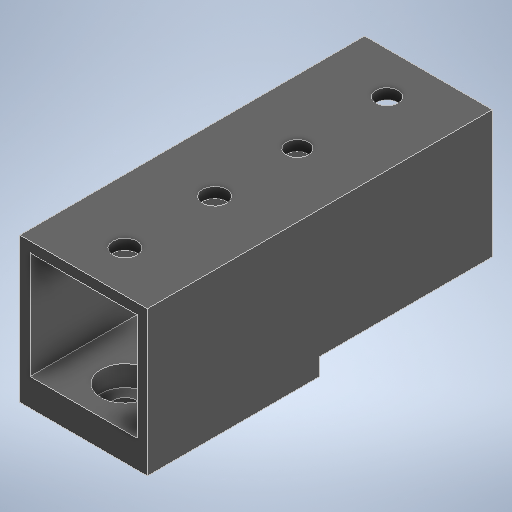
# Autodesk Inventor part: pole_setter_arm
Saved by Autodesk Inventor 2026.1 (Build 301233020, 233B)
## iProperties
Created: 2026-02-01
Part Number: pole_setter_arm
Material: 一般
Document SubType Name: Modeling
Designer: hibik
Density: 1 g/cm^3
Appearance: 既定
Author: hibik
Autodesk Inventor part; units mm, degrees
ref_plane "YZ Plane" through (0, 0, 0) normal (1, 0, 0) x (0, 1, 0)
ref_plane "XZ Plane" through (0, 0, 0) normal (0, 1, 0) x (-1, 0, 0)
ref_plane "XY Plane" through (0, 0, 0) normal (0, 0, 1) x (1, 0, 0)
sketch "スケッチ1" plane through (0, 0, 0) normal (0, 1, 0) x (-1, 0, 0)
  line L0 (0, 12.5) -> (18.5, 12.5)
  line L1 (18.5, 12.5) -> (18.5, -12.5)
  line L2 (18.5, -12.5) -> (0, -12.5)
  line L3 (0, -12.5) -> (0, 12.5)
  point P0 (0, 0)
  point P1 (0, 0)
  dimension "d0" = 18.5
  dimension "d1" = 25
  constraints: 8 end point, 2 parallel, 1 coincident, 1 horizontal, 1 midpoint, 1 perpendicular
  measures "d0" distance of L1.end L2.end
  measures "d1" distance of L0.end L1.end
extrude "押し出し1" add sketch "スケッチ1" along normal blind 1
sketch "スケッチ3" plane through (0, 1, 0) normal (0, 1, 0) x (1, 0, 0)
  circle A0 centre (-9.25, -6.5) radius 1.75
  circle A1 centre (-9.25, 6.5) radius 1.75
  line L0 (-22.2, 0) -> (3.7, 0) projected
  line L1 (-18.5, -12.5) -> (0, -12.5) projected
  point P0 (0, 0)
  point P1 (-9.25, -12.5)
  dimension "d9" = 6
  dimension "d10" = 3.5
  constraints: 2 centre point, 1 midpoint, 1 vertical alignment, 1 other
  measures "d9" distance from line of L1 A0.centre
  measures "d10" diameter of A0
extrude "押し出し3" cut sketch "スケッチ3" against normal through all
sketch "スケッチ4" plane through (0, 1, 0) normal (0, 1, 0) x (1, 0, 0)
  circle A0 centre (-9.25, -6.5) radius 1.75 projected
  circle A1 centre (-9.25, 6.5) radius 1.75 projected
  line L0 (0, 12.5) -> (-18.5, 12.5) projected
  line L1 (-18.5, 12.5) -> (-18.5, -12.5) projected
  line L2 (-18.5, -12.5) -> (0, -12.5) projected
  line L3 (0, -12.5) -> (0, 12.5) projected
  circle A2 centre (-9.25, 6.5) radius 3.5
  circle A3 centre (-9.25, -6.5) radius 3.5
  point P0 (0, 0)
  dimension "d13" = 7
  dimension "d14" = 7
  constraints: 2 centre point, 2 coincident
  measures "d13" diameter of A2
  measures "d14" diameter of A3
extrude "押し出し4" add sketch "スケッチ4" along normal blind 1.5 contours L3 L2 L1 L0
sketch "スケッチ5" plane through (-18.5, 0, 12.5) normal (0, 0, 1) x (1, 0, 0)
  line L0 (0, 2.5) -> (18.5, 2.5)
  line L1 (18.5, 2.5) -> (18.5, 21)
  line L2 (18.5, 21) -> (0, 21)
  line L3 (0, 21) -> (0, 2.5)
  line L4 (1.5, 4) -> (17, 4)
  line L5 (17, 4) -> (17, 19.5)
  line L6 (17, 19.5) -> (1.5, 19.5)
  line L7 (1.5, 19.5) -> (1.5, 4)
  point P0 (18.5, 0)
  point P1 (9.25, 19.5)
  point P2 (9.25, 21)
  dimension "d17" = 1.5
  dimension "d18" = 1.5
  dimension "d19" = 15.5
  constraints: 16 end point, 4 parallel, 4 perpendicular, 2 horizontal, 2 midpoint, 1 coincident, 1 vertical alignment
  measures "d17" distance between parallel lines of L2 L6
  measures "d18" distance between parallel lines of L7 L3
  measures "d19" distance of L4.end L5.end
extrude "押し出し5" add sketch "スケッチ5" against normal up to surface (25 mm away)
sketch "スケッチ6" plane through (-17, 4, 12.5) normal (0, 1, 0) x (1, 0, 0)
  circle A0 centre (7.75, 6) radius 3.5 projected
  circle A1 centre (7.75, 19) radius 3.5 projected
  point P0 (17, 12.5)
extrude "押し出し6" cut sketch "スケッチ6" against normal up to surface (1.5 mm away)
sketch "スケッチ7" plane through (-18.5, 21, 12.5) normal (0, 1, 0) x (1, 0, 0)
  circle A0 centre (9.25, 19) radius 1.75 projected
  circle A1 centre (9.25, 6) radius 1.75 projected
  point P0 (18.5, 12.5)
extrude "押し出し7" cut sketch "スケッチ7" against normal through all
sketch "スケッチ9" plane through (0, 0, -12.5) normal (0, 0, -1) x (-1, 0, 0)
  line L0 (0, 0) -> (0, 21) projected
  line L1 (18.5, 0) -> (18.5, 21) projected
  line L2 (0, 2.5) -> (18.5, 2.5)
  line L3 (18.5, 2.5) -> (18.5, 21)
  line L4 (18.5, 21) -> (0, 21)
  line L5 (0, 21) -> (0, 2.5)
  line L6 (1.5, 4) -> (17, 4) projected
  line L7 (1.5, 19.5) -> (1.5, 4) projected
  line L8 (17, 19.5) -> (1.5, 19.5) projected
  line L9 (17, 4) -> (17, 19.5) projected
  dimension "d32" = 18.5
  constraints: 8 end point, 2 parallel, 1 horizontal, 1 perpendicular, 1 point on line
  measures "d32" distance between parallel lines of L2 L4
extrude "押し出し9" add sketch "スケッチ9" along normal blind 25
sketch "スケッチ10" plane through (-18.5, 21, 12.5) normal (0, 1, 0) x (1, 0, 0)
  circle A0 centre (9.25, 44) radius 1.6
  circle A1 centre (9.25, 31) radius 1.6
  line L0 (0, 50) -> (18.5, 50) projected
  point P0 (18.5, 12.5)
  point P1 (9.25, 50)
  dimension "d35" = 3.2
  dimension "d36" = 3.2
  dimension "d37" = 6
  dimension "d38" = 13
  constraints: 2 centre point, 2 vertical alignment, 1 midpoint
  measures "d35" diameter of A0
  measures "d36" diameter of A1
  measures "d37" distance from line of L0 A0.centre
  measures "d38" distance of A1.centre A0.centre
extrude "押し出し10" cut sketch "スケッチ10" against normal through all
equation "\"d18\" = d17"
